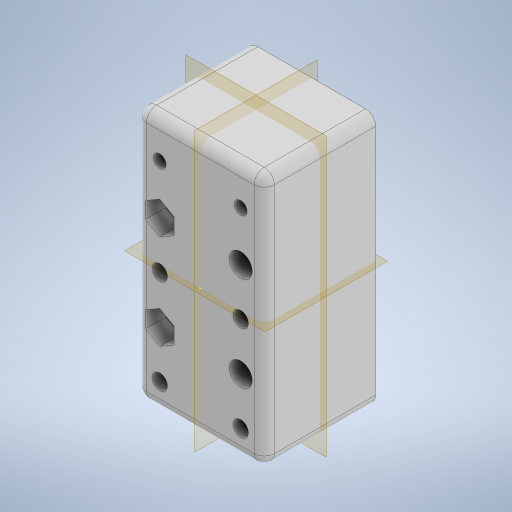
# Autodesk Inventor part: крепление петли хвоста
Saved by Autodesk Inventor 2023.2 (Build 272271030, 271C)
## iProperties
Created: 2024-03-15
Part Number: крепление петли хвоста
Material: Типовые
Document SubType Name: Modeling
Designer: I9232
Density: 1 g/cm^3
Appearance: По умолчанию
Author: I9232
Autodesk Inventor part; units mm, degrees
sketch "Эскиз1" plane through (0, 0, 0) normal (0, 0, 1) x (1, 0, 0)
  line L0 (-12.625, -25) -> (12.625, -25)
  line L1 (12.625, -25) -> (12.625, 25)
  line L2 (12.625, 25) -> (-12.625, 25)
  line L3 (-12.625, 25) -> (-12.625, -25)
  line L4 (-12.625, -25) -> (12.625, 25) construction
  line L5 (12.625, -25) -> (-12.625, 25) construction
  point P0 (0, 0)
  dimension "d0" = 25.25
  dimension "d1" = 50
  constraints: 12 end point, 2 midpoint, 2 parallel, 1 horizontal, 1 perpendicular
  measures "d0" distance of L1.end L2.end
  measures "d1" distance of L0.end L1.end
extrude "Выдавливание1" add sketch "Эскиз1" along normal mid plane 22
fillet "Сопряжение1" radius 2 8 edges at (-12.625, -25, 0) (0, -25, 11) (-12.625, 0, 11) (12.625, 0, 11) (12.625, -25, 0) (0, 25, 11) (12.625, 25, 0) (-12.625, 25, 0)
sketch "Эскиз2" plane through (0, 0, 11) normal (0, 0, 1) x (1, 0, 0)
  circle A0 centre (-8, 17.75) radius 1.25
  circle A1 centre (8, 17.75) radius 1.25
  line L0 (-10.625, 23) -> (10.625, 23) projected
  point P0 (0, 0)
  dimension "d17" = 5.25
  dimension "d18" = 5.25
  constraints: 2 centre point
  measures "d17" distance from line of L0 A0.centre
  measures "d18" distance from line of A1.centre L0
extrude "Выдавливание2" cut sketch "Эскиз2" against normal up to surface (22 mm away)
sketch "Эскиз3" plane through (0, 0, 11) normal (0, 0, 1) x (1, 0, 0)
  point P0 (0, 0)
sketch "Эскиз4" plane through (0, 0, 11) normal (0, 0, 1) x (1, 0, 0)
  circle A0 centre (8, 8) radius 1.5
  circle A1 centre (-8, 8) radius 1.5
  line L0 (-8, 8) -> (8, 8) construction
  circle A2 centre (-8, 17.75) radius 1.25 construction
  line L1 (-8, 17.75) -> (-8, 4.7032) construction
  line L2 (10.625, -23) -> (-10.625, -23) construction
  point P0 (0, 0)
  dimension "d7" = 3
  dimension "d8" = 16
  dimension "d16" = 9.75
  constraints: 4 end point, 2 centre point, 1 equal radius, 1 horizontal, 1 point on line, 1 vertical
  measures "d7" diameter of A0
  measures "d8" distance of L0.start L0.end
  measures "d16" distance of L1.start L0.start
extrude "Выдавливание3" cut sketch "Эскиз4" against normal up to surface (22 mm away)
sketch "Эскиз5" plane through (0, 0, 11) normal (0, 0, 1) x (1, 0, 0)
  circle A0 centre (8, 8) radius 1.5 projected
  circle A1 centre (8, 8) radius 2.25
  circle A2 centre (-8, 8) radius 1.5 projected
  line L0 (-8, 11.2332) -> (-5.2, 9.6166)
  line L1 (-5.2, 9.6166) -> (-5.2, 6.3834)
  line L2 (-5.2, 6.3834) -> (-8, 4.7668)
  line L3 (-8, 4.7668) -> (-10.8, 6.3834)
  line L4 (-10.8, 6.3834) -> (-10.8, 9.6166)
  line L5 (-10.8, 9.6166) -> (-8, 11.2332)
  point P0 (0, 0)
  dimension "d12" = 4.5
  dimension "d15" = 5.6
  constraints: 12 end point, 2 coincident, 1 centre point, 13 other
  measures "d12" diameter of A1
  measures "d15" distance between parallel lines of L4 L1
extrude "Выдавливание4" cut sketch "Эскиз5" against normal blind 4
sketch "Эскиз6" plane through (0, 0, 11) normal (0, 0, 1) x (1, 0, 0)
  circle A0 centre (-8, -1.3) radius 1.5
  circle A1 centre (8, -1.3) radius 1.5
  circle A2 centre (-8, -20) radius 1.5
  circle A3 centre (8, -20) radius 1.5
  line L0 (-8, -1.3) -> (-8, -20) construction
  line L1 (-8, -1.3) -> (8, -1.3) construction
  line L2 (-8, -20) -> (8, -20) construction
  line L3 (-10.625, -25) -> (10.625, -25) projected
  line L4 (10.625, -23) -> (-10.625, -23) projected
  line L5 (0, -23) -> (0, 23) construction
  line L6 (-10.625, 23) -> (10.625, 23) projected
  line L7 (0, 35) -> (0, -35) projected
  circle A4 centre (-8, 8) radius 1.5 projected
  point P0 (0, 0)
  point P1 (0, -20)
  dimension "d19" = 3
  dimension "d20" = 16
  dimension "d21" = 16
  dimension "d23" = 5
  dimension "d40" = 9.3
  constraints: 8 end point, 4 centre point, 3 coincident, 3 equal radius, 3 midpoint, 2 horizontal, 1 point on line, 1 vertical
  measures "d19" diameter of A0
  measures "d20" distance of A1.centre L0.start
  measures "d21" distance of A3.centre A2.centre
  measures "d23" distance from line of L3 A2.centre
  measures "d40" distance of A4.centre L0.start
extrude "Выдавливание5" cut sketch "Эскиз6" against normal blind 5 contours A0 | A1 | A2 | A3
sketch "Эскиз7" plane through (0, 0, 11) normal (0, 0, 1) x (1, 0, 0)
  circle A0 centre (-8, -20) radius 1.5 projected
  circle A1 centre (-8, -1.3) radius 1.5 projected
  line L0 (-8, -20) -> (-8, -1.3) construction
  circle A2 centre (8, -20) radius 1.5 projected
  circle A3 centre (8, -1.3) radius 1.5 projected
  line L1 (8, -20) -> (8, -1.3) construction
  circle A4 centre (8, -10.7) radius 2.25
  line L2 (-10.8, -9.0834) -> (-8, -7.4668)
  line L3 (-8, -7.4668) -> (-5.2, -9.0834)
  line L4 (-5.2, -9.0834) -> (-5.2, -12.3166)
  line L5 (-5.2, -12.3166) -> (-8, -13.9332)
  line L6 (-8, -13.9332) -> (-10.8, -12.3166)
  line L7 (-10.8, -12.3166) -> (-10.8, -9.0834)
  circle A5 centre (-8, -10.7) radius 1.5
  circle A6 centre (8, -10.7) radius 1.5
  point P0 (0, 0)
  dimension "d28" = 4.5
  dimension "d29" = 5.6
  dimension "d35" = 3
  dimension "d41" = 9.3
  dimension "d42" = 9.3
  constraints: 16 end point, 3 centre point, 2 coincident, 2 vertical, 1 equal radius, 13 other
  measures "d28" diameter of A4
  measures "d29" distance between parallel lines of L4 L7
  measures "d35" diameter of A5
  measures "d41" distance of L0.start point (-8, -10.7)
  measures "d42" distance of L1.start A4.centre
extrude "Выдавливание8" cut sketch "Эскиз7" against normal blind 4 contours A4 | L2 L3 L4 L5 L6 L7
sketch "Эскиз9" plane through (0, 0, 11) normal (0, 0, 1) x (1, 0, 0)
  circle A0 centre (-8, -10.7) radius 1.5 projected
  circle A1 centre (8, -10.7) radius 1.5 projected
  point P0 (0, 0)
extrude "Выдавливание9" cut sketch "Эскиз9" against normal up to surface (22 mm away)
